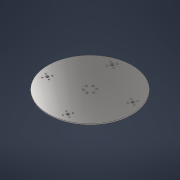
# Autodesk Inventor part: support disk-2
Saved by Autodesk Inventor 2021 (Build 250183000, 183)
## iProperties
Created: 2021-02-20
Part Number: support disk-2
Material: Steel, Mild
Document SubType Name: Modeling
Designer: vikki
Density: 7.85 g/cm^3
Appearance: Semi-Polished
Author: vikki
Autodesk Inventor part; units mm, degrees
ref_plane "YZ Plane" through (0, 0, 0) normal (1, 0, 0) x (0, 1, 0)
ref_plane "XZ Plane" through (0, 0, 0) normal (0, 1, 0) x (-1, 0, 0)
ref_plane "XY Plane" through (0, 0, 0) normal (0, 0, 1) x (1, 0, 0)
sketch "Sketch1" plane through (0, 0, 0) normal (0, 1, 0) x (-1, 0, 0)
  circle A0 centre (0, 0) radius 136
  dimension "d0" = 272
  constraints: 1 centre point, 1 coincident
  measures "d0" diameter of A0
extrude "Extrusion1" add sketch "Sketch1" along normal blind 3
sketch "Sketch2" plane through (0, 3, 0) normal (0, 1, 0) x (1, 0, 0)
  circle A0 centre (-110.2956, -43.8634) radius 1.85 projected
  circle A1 centre (-115.3836, -27.8523) radius 1.85 projected
  circle A2 centre (-94.2846, -38.7754) radius 1.85 projected
  circle A3 centre (-99.3725, -22.7644) radius 1.85 projected
  circle A4 centre (-43.8634, 110.2956) radius 1.85 projected
  circle A5 centre (-27.8523, 115.3836) radius 1.85 projected
  circle A6 centre (-38.7754, 94.2846) radius 1.85 projected
  circle A7 centre (-22.7644, 99.3725) radius 1.85 projected
  circle A8 centre (110.2956, 43.8634) radius 1.85 projected
  circle A9 centre (115.3836, 27.8523) radius 1.85 projected
  circle A10 centre (94.2846, 38.7754) radius 1.85 projected
  circle A11 centre (99.3725, 22.7644) radius 1.85 projected
  circle A12 centre (43.8634, -110.2956) radius 1.85 projected
  circle A13 centre (27.8523, -115.3836) radius 1.85 projected
  circle A14 centre (38.7754, -94.2846) radius 1.85 projected
  circle A15 centre (22.7644, -99.3725) radius 1.85 projected
  circle A16 centre (104.8341, 33.3139) radius 4 projected
  circle A17 centre (-104.8341, -33.3139) radius 4 projected
  circle A18 centre (-33.3139, 104.8341) radius 4 projected
  circle A19 centre (33.3139, -104.8341) radius 4 projected
  circle A20 centre (0, 0) radius 135 projected
  circle A21 centre (-14.6517, 3.2136) radius 2.5 projected
  circle A22 centre (-4.5428, 14.2956) radius 2.5 projected
  circle A23 centre (10.1089, 11.082) radius 2.5 projected
  circle A24 centre (14.6517, -3.2136) radius 2.5 projected
  circle A25 centre (4.5428, -14.2956) radius 2.5 projected
  circle A26 centre (-10.1089, -11.082) radius 2.5 projected
  point P0 (0, 0)
extrude "Extrusion2" cut sketch "Sketch2" against normal up to surface (3 mm away) contours A0 | A1 | A2 | A3 | A4 | A5 | A6 | A7 | A8 | A9 | A10 | A11 | A12 | A13 | A14 | A15 | A16 | A17 | A18 | A19 | A21 | A22 | A23 | A24 | A25 | A26
body "Solid1"
